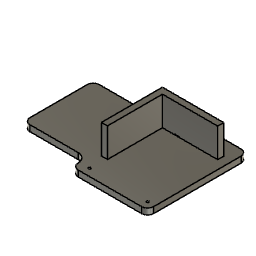
FSRMountPioneer v4 (Autodesk Fusion 360 design; units mm, degrees)
Autodesk Fusion 360 part; units mm, degrees
note: some values were not read from the file. Set by a fixed rule: which sketch regions a step uses; which face or edge a step refers to.
sketch "Sketch1" plane through (0, 0, 0) normal (0, 0, 1) x (1, 0, 0)
  line L0 (0, 0) -> (-60, 0)
  line L1 (-60, 0) -> (-60, -90)
  line L2 (60, 0) -> (60, 90)
  line L3 (-60, -90) -> (60, -90)
  line L4 (60, -90) -> (60, 90)
  line L5 (60, 90) -> (-60, 90)
  line L6 (-60, 90) -> (-60, -90)
  line L7 (0, -90) -> (0, -75)
  line L8 (0, -90) -> (0, -71)
  line L9 (0, -75) -> (0, -73)
  line L10 (0, -73) -> (-48, -73)
  line L11 (0, -73) -> (48, -73)
  circle A0 centre (-48, -73) radius 2
  circle A1 centre (48, -73) radius 2
  line L12 (0, -90) -> (0, 68)
  circle A2 centre (0, 68) radius 2
  dimension "d4" = 60
  dimension "d5" = 60
  dimension "d6" = 90
  dimension "d8" = 90
  dimension "d9" = 15
  dimension "d10" = 48
  dimension "d11" = 48
  dimension "d13" = 4
  dimension "d14" = 4
  dimension "d15" = 158
  dimension "d16" = 4
  constraint coincident L0.start origin
  constraint horizontal L0
  constraint perpendicular L0 L1
  constraint horizontal L3
  constraint vertical L4
  constraint horizontal L5
  constraint vertical L6
  constraint midpoint L3 L7.start
  constraint perpendicular L3 L7
  constraint perpendicular L3 L8
  constraint coincident L8 L9.end
  constraint parallel L8 L9
  constraint perpendicular L9 L10
  constraint perpendicular L8 L11
  constraint coincident L10.end A0.centre
  constraint coincident L11.end A1.centre
  constraint parallel L8 L12
  constraint coincident L12.end A2.centre
  measures "d4" distance of L0.start L0.end
  measures "d5" distance of L0.start L2.start
  measures "d6" distance of L0.end L1.end
  measures "d8" distance of L2.start L2.end
  measures "d9" distance of L7.start L7.end
  measures "d10" distance of L9.end L10.end
  measures "d11" distance of L9.end L11.end
  measures "d13" diameter of A0
  measures "d14" diameter of A1
  measures "d15" distance of L7.start L12.end
  measures "d16" diameter of A2
extrude "Extrude1" add sketch "Sketch1" along normal blind 10 makes body 1
move_face "OffsetFaces1" offset -5 1 faces at (-40, -90, 3.3333) on bodies 1
fillet "Fillet2" radius 10 1 edges at (60, -85, 5) on bodies 1
sketch "Sketch2" plane through (0, 0, 10) normal (0, 0, 1) x (-1, 0, 0)
  line L0 (60, -90) -> (60, 85)
  line L1 (60, 85) -> (-50, 85)
  arc A0 (-50, 85) -> (-60, 75) centre (-50, 75) ccw
  line L2 (-60, 75) -> (-60, -90)
  line L3 (-60, -90) -> (60, -90)
  circle A1 centre (48, 73) radius 2
  circle A2 centre (-48, 73) radius 2
  circle A3 centre (0, -68) radius 2
  line L4 (0, 0) -> (43.7, 0)
  line L5 (43.7, 0) -> (43.7, -43.7)
  line L6 (43.7, -43.7) -> (0, -43.7)
  line L7 (0, -43.7) -> (0, 0)
  line L8 (0, 0) -> (-43.7, 0)
  line L9 (-43.7, 0) -> (-43.7, -43.7)
  line L10 (-43.7, -43.7) -> (0, -43.7)
  line L11 (0, -43.7) -> (0, 0)
  line L12 (-43.7, -43.7) -> (44.2, -43.7)
  line L13 (44.2, -43.7) -> (44.2, 43.7)
  line L14 (44.2, 43.7) -> (-43.7, 43.7)
  line L15 (-43.7, 43.7) -> (-43.7, -43.7)
  line L16 (0, 0) -> (0, 43.7)
  line L17 (-45.5, -45.5) -> (46, -45.5)
  line L18 (46, -45.5) -> (46, 45.5)
  line L19 (46, 45.5) -> (-45.5, 45.5)
  line L20 (-45.5, 45.5) -> (-45.5, -45.5)
  line L21 (-45.5, -45.5) -> (-45.5, -55.5)
  line L22 (-45.5, -55.5) -> (45.5, -55.5)
  line L23 (56, -45.5) -> (56, -55.5)
  line L24 (56, -55.5) -> (45.5, -55.5)
  line L25 (46, 45.5) -> (56, 45.5)
  line L26 (56, 45.5) -> (56, -45.5)
  line L27 (21.85, -43.7) -> (21.85, -55.5)
  line L28 (21.85, -43.7) -> (25.85, -43.7)
  line L29 (25.85, -43.7) -> (17.85, -43.7)
  line L30 (17.85, -43.7) -> (17.85, -55.5)
  line L31 (17.85, -55.5) -> (25.85, -55.5)
  line L32 (25.85, -55.5) -> (25.85, -43.7)
  line L33 (25.85, -43.7) -> (25.85, -45.5)
  line L34 (17.85, -45.5) -> (17.85, -43.7)
  dimension "d28" = 43.7
  dimension "d29" = 43.7
  dimension "d30" = 43.7
  dimension "d31" = 43.7
  dimension "d33" = 87.4
  dimension "d34" = 43.7
  dimension "d35" = 1.8
  dimension "d38" = 10
  dimension "d39" = 10
  dimension "d40" = 10
  dimension "d41" = 4
  dimension "d42" = 8
  constraint horizontal L4
  constraint vertical L5
  constraint horizontal L6
  constraint vertical L7
  constraint coincident L4.start L7.end
  constraint horizontal L8
  constraint vertical L9
  constraint horizontal L10
  constraint vertical L11
  constraint horizontal L12
  constraint vertical L13
  constraint horizontal L14
  constraint vertical L15
  constraint perpendicular L4 L16
  constraint perpendicular L17 L21
  constraint perpendicular L18 L25
  constraint perpendicular L25 L26
  constraint midpoint L6 L27.start
  constraint coincident L22 L27.end
  constraint perpendicular L22 L27
  constraint perpendicular L27 L28
  constraint horizontal L29
  constraint vertical L30
  constraint horizontal L31
  constraint vertical L32
  constraint coincident L32 L33.end
  constraint coincident L17 L33.end
  constraint coincident L17 L34.start
  constraint coincident L30 L34.start
  measures "d28" distance of L4.start L4.end
  measures "d29" distance of L4.start L6.end
  measures "d30" distance of L4.start L8.end
  measures "d31" distance of L4.start L6.end
  measures "d33" distance of L9.end L14.end
  measures "d34" distance of L4.start L16.end
  measures "d38" distance of L17.start L21.end
  measures "d39" distance of L17.end L23.start
  measures "d40" distance of L18.end L25.end
  measures "d41" distance of L27.start L28.end
  measures "d42" distance of L28.end L29.end
copy_body "CutPasteBodies1" bodies 1 removing the originals makes body 2 in component "Base"
extrude "Extrude1'" cut sketch "Sketch2" against normal blind 5 contours L17 L21 L22 L30 | L17 L22 L27 L30 L31 | L17 L22 L27 L31 L32 | L17 L18 L22 L23 L24 L25 L26 L32 bodies 2 in component "Base"
extrude "Extrude2" add 1 faces at (-60, 31.6667, 3.3333) along direction (-1, 0, 0) blind 110 on bodies 2 bodies 2 in component "Base"
extrude "Extrude3" cut 1 faces at (-93.3333, 90, 3.3333) along direction (0, -1, 0) blind 10 on bodies 2 bodies 2 in component "Base"
fillet "Fillet1" radius 10 1 edges at (60, 80, 5) on bodies 2 in component "Base"
sketch "Sketch2 (2)" plane through (0, 80, 0) normal (0, 1, 0) x (-1, 0, 0) in component "Base"
  line L0 (-50, 10) -> (-50, 0)
  line L1 (-50, 0) -> (170, 0)
  line L2 (170, 0) -> (170, 10)
  line L3 (170, 10) -> (-50, 10)
  line L4 (170, 10) -> (65, 10)
  line L5 (65, 10) -> (65, 0)
  dimension "d51" = 105
  constraint coincident L2.end L3.start
  constraint perpendicular L2 L4
  constraint coincident L1 L5.end
  constraint perpendicular L1 L5
  measures "d51" distance of L2.end L4.end
extrude "Extrude4" cut sketch "Sketch2 (2)" against normal blind 25 contours L1 L2 L3 L4 L5 bodies 2 in component "Base"
sketch "Sketch3" plane through (0, -85, 0) normal (0, -1, 0) x (1, 0, 0) in component "Base"
  line L0 (50, 0) -> (50, 10)
  line L1 (50, 10) -> (-170, 10)
  line L2 (-170, 10) -> (-170, 0)
  line L3 (-170, 0) -> (50, 0)
  line L4 (-170, 10) -> (-65, 10)
  line L5 (-65, 10) -> (-65, 0)
  dimension "d54" = 105
  constraint coincident L1.end L2.start
  constraint perpendicular L2 L4
  constraint coincident L3 L5.end
  constraint perpendicular L3 L5
  measures "d54" distance of L1.end L4.end
extrude "Extrude5" cut sketch "Sketch3" against normal blind 25 contours L1 L2 L3 L4 L5 bodies 2 in component "Base"
fillet "Fillet2'" radius 10 1 edges at (-170, -60, 5) on bodies 2 in component "Base"
fillet "Fillet3" radius 10 1 edges at (-170, 55, 5) on bodies 2 in component "Base"
fillet "Fillet4" radius 10 1 edges at (-65, -85, 5) on bodies 2 in component "Base"
fillet "Fillet5" radius 10 1 edges at (-65, 80, 5) on bodies 2 in component "Base"
fillet "Fillet6" radius 15 1 edges at (-65, 55, 5) on bodies 2 in component "Base"
fillet "Fillet7" radius 15 1 edges at (-65, -60, 5) on bodies 2 in component "Base"
extrude "Extrude1''" add sketch "Sketch2" along normal blind 48 separate body contours L17 L21 L22 L30 | L17 L22 L27 L30 L31 | L17 L22 L27 L31 L32 | L17 L18 L22 L23 L24 L25 L26 L32 makes body 3 in component "Wall"
extrude "Extrude2'" cut sketch "Sketch2" along normal blind 1 contours L17 L22 L27 L30 L31 | L17 L22 L27 L31 L32 bodies 3 in component "Wall"
extrude "Extrude3'" add sketch "Sketch2" against normal blind 5 contours L17 L21 L22 L30 | L17 L18 L22 L23 L24 L25 L26 L32 bodies 3 in component "Wall"
sketch "Sketch4" plane through (0, 0, 10) normal (0, 0, 1) x (-1, 0, 0) in component "Base"
  arc A0 (55, -80) -> (65, -70) centre (55, -70) ccw
  arc A1 (80, -55) -> (65, -70) centre (80, -70) ccw
  line L0 (80, -55) -> (160, -55)
  arc A2 (160, -55) -> (170, -45) centre (160, -45) ccw
  line L1 (170, -45) -> (170, 50)
  arc A3 (170, 50) -> (160, 60) centre (160, 50) ccw
  line L2 (160, 60) -> (80, 60)
  arc A4 (65, 75) -> (80, 60) centre (80, 75) ccw
  arc A5 (65, 75) -> (55, 85) centre (55, 75) ccw
  line L3 (55, 85) -> (-50, 85)
  arc A6 (-50, 85) -> (-60, 75) centre (-50, 75) ccw
  line L4 (-60, 75) -> (-60, -70)
  arc A7 (-60, -70) -> (-50, -80) centre (-50, -70) ccw
  line L5 (-50, -80) -> (55, -80)
  line L6 (56, -55.5) -> (-45.5, -55.5)
  line L7 (-45.5, -55.5) -> (-45.5, -45.5)
  line L8 (-45.5, -45.5) -> (46, -45.5)
  line L9 (46, -45.5) -> (46, 45.5)
  line L10 (46, 45.5) -> (56, 45.5)
  line L11 (56, 45.5) -> (56, -55.5)
  circle A8 centre (48, 73) radius 2
  circle A9 centre (-48, 73) radius 2
  circle A10 centre (0, -68) radius 2
  line L12 (-45.625, -45.375) -> (45.875, -45.375)
  line L13 (45.875, -45.375) -> (45.875, 45.625)
  line L14 (45.875, 45.625) -> (56.125, 45.625)
  line L15 (56.125, 45.625) -> (56.125, -55.625)
  line L16 (56.125, -55.625) -> (-45.625, -55.625)
  line L17 (-45.625, -55.625) -> (-45.625, -45.375)
extrude "Extrude6" cut sketch "Sketch4" against normal up to surface (5 mm away) contours L12 L13 L14 L15 L16 L17 bodies 2 in component "Base"
component "Base" placed x (1, 0, 0) y (0, 1, 0) z (0, 0, 1) at (0, 0, 0)
component "Wall" placed x (1, 0, 0) y (0, 1, 0) z (0, 0, 1) at (0, 0, 0)
equation "tolerance = 0.125 mm"
equation "d76 = -tolerance"
